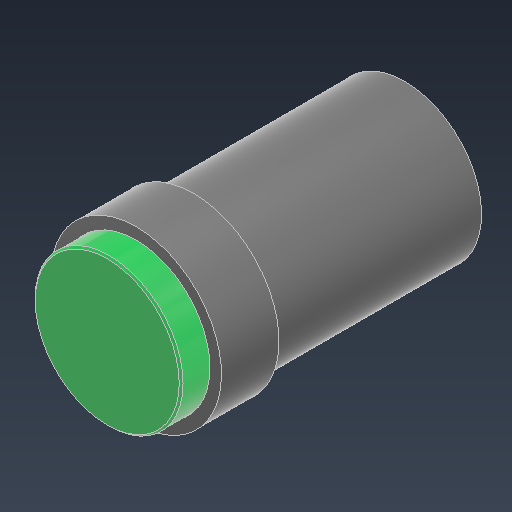
# Autodesk Inventor part: AP6MS54G
Saved by Autodesk Inventor 2021 (Build 250183000, 183)
## iProperties
Created: 2021-07-24
Part Number: AP6MS54G
Material: ABS プラスチック
Document SubType Name: Modeling
Designer: yuta0
Density: 1.06 g/cm^3
Appearance: 滑らか - 黒
Description: Amazon
購入先: Amazon
在庫数: 0.0
Author: yuta0
Autodesk Inventor part; units mm, degrees
ref_plane "YZ Plane" through (0, 0, 0) normal (1, 0, 0) x (0, 1, 0)
ref_plane "XZ Plane" through (0, 0, 0) normal (0, 1, 0) x (-1, 0, 0)
ref_plane "XY Plane" through (0, 0, 0) normal (0, 0, 1) x (1, 0, 0)
sketch "スケッチ1" plane through (0, 0, 0) normal (1, 0, 0) x (0, 1, 0)
  line L0 (8.9, -3) -> (8.9, -9)
  line L1 (8.9, -9) -> (8, -9)
  line L2 (8, -9) -> (8, -31)
  line L3 (8, -31) -> (0, -31)
  line L4 (0, -31) -> (0, 0)
  line L5 (8.9, -3) -> (7.7, -3)
  line L6 (7.7, -3) -> (7.7, 0)
  line L7 (7.7, 0) -> (0, 0)
  dimension "d0" = 8.9
  dimension "d1" = 3
  dimension "d2" = 9
  dimension "d3" = 31
  dimension "d4" = 7.7
  dimension "d5" = 8
  constraints: 16 end point, 7 perpendicular, 1 horizontal
  measures "d0" distance between parallel lines of L4 L0
  measures "d1" distance of L5.end L6.end
  measures "d2" distance between parallel lines of L7 L1
  measures "d3" distance of L3.end L4.end
  measures "d4" distance of L6.end L4.end
  measures "d5" distance between parallel lines of L4 L2
revolve "回転1" add sketch "スケッチ1" angle 360 about axis through (0, 0, -31) along (0, 0, 1)
chamfer "面取り1" distance 0.2 angle 45 1 edges at (0, -7.7, 0)
